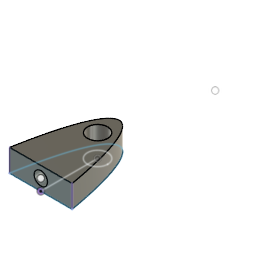
stand (Autodesk Fusion 360 design; units mm, degrees)
part number: 2026-05-16-13-36-09-103
Autodesk Fusion 360 part; units mm, degrees
note: some values were not read from the file. Set by a fixed rule: which sketch regions a step uses.
sketch "Sketch1" plane through (0, 0, 0) normal (0, 0, 1) x (1, 0, 0)
  line L0 (0, 0) -> (0, 12.7)
  circle A0 centre (0, 12.7) radius 2.25
  line L1 (-7, 0) -> (7, 0)
  spline S0 degree 2 poles (7, 0) (0, 39) (-7, 0) knots 0 0 0 3.778902 3.778902 3.778902 weights 1 0.818182 1
  dimension "d1" = 12.7
  dimension "d3" = 4.5
  constraint coincident L0.start origin
  constraint vertical L0
  constraint coincident L0.end A0.centre
  constraint perpendicular L0 L1
  measures "d1" distance of L0.start L0.end
  measures "d3" diameter of A0
extrude "Extrude1" add sketch "Sketch1" along normal blind 5
sketch "Sketch2" plane through (0, 0, 0) normal (0, -1, 0) x (1, 0, 0)
  line L0 (-7, 0) -> (7, 0)
  line L1 (7, 5) -> (-7, 5)
  line L2 (7, 0) -> (7, 5)
  line L3 (-7, 5) -> (-7, 0)
  point P0 (0, 2.5)
hole "Hole1" at (0, 0, 2.5) direction (0, 1, 0) diameter 3 depth 5 tip angle 180
